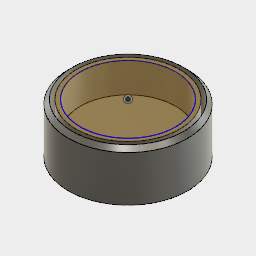
ANS0013_moving_bottom v3 (Autodesk Fusion 360 design; units mm, degrees)
Autodesk Fusion 360 part; units mm, degrees
sketch "Sketch1" plane through (0, 0, 0) normal (0, 1, 0) x (1, 0, 0)
  circle A0 centre (0, 0) radius 30
  dimension "d1" = 60
  measures "d1" diameter of A0
extrude "Extrude1" add sketch "Sketch1" along normal blind 25
sketch "Sketch2" plane through (0, 25, 0) normal (0, 1, 0) x (-1, 0, 0)
  circle A0 centre (0, 0) radius 30
  circle A1 centre (0, 0) radius 28
  circle A2 centre (0, 0) radius 26
  circle A3 centre (0, 0) radius 24
  dimension "d4" = 56
  dimension "d5" = 52
  dimension "d6" = 48
  measures "d4" diameter of A1
  measures "d5" diameter of A2
  measures "d6" diameter of A3
extrude "Extrude2" cut sketch "Sketch2" against normal blind 15 contours A1
sketch "Sketch3" plane through (0, 25, 0) normal (0, 1, 0) x (-1, 0, 0)
  circle A0 centre (0, 0) radius 26
  circle A1 centre (0, 0) radius 24
  dimension "d9" = 48
  measures "d9" diameter of A1
extrude "Extrude3" cut sketch "Sketch3" against normal blind 15 contours A1
extrude "Extrude4" cut sketch "Sketch3" against normal blind 15 contours A1
chamfer "Chamfer1" distance 2 angle 45 1 edges at (-27.9698, 25, 10.8485)
